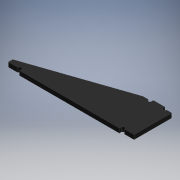
# Autodesk Inventor part: 前腕_サブフレーム_1_1
Saved by Autodesk Inventor 2018 (Build 220112000, 112)
## iProperties
Created: 2016-05-04
Part Number: 前腕_サブフレーム_1_1
Material: アセタール樹脂、黒
Document SubType Name: Modeling
Designer: hiroaki
Density: 1.425 g/cm^3
Appearance: 滑らか - 黒
Mass: 16.6655 g
Surface Area: 81.5563 cm^2
Volume: 11.6951 cm^3
Author: hiroaki
Autodesk Inventor part; units mm, degrees
ref_plane "YZ Plane" through (0, 0, 0) normal (1, 0, 0) x (0, 1, 0)
ref_plane "XZ Plane" through (0, 0, 0) normal (0, 1, 0) x (-1, 0, 0)
ref_plane "XY Plane" through (0, 0, 0) normal (0, 0, 1) x (1, 0, 0)
sketch "スケッチ1" plane through (0, 0, 0) normal (0, 0, 1) x (1, 0, 0)
  line L0 (-72.5, -21.65) -> (72.5, -21.65) construction
  line L1 (72.5, -21.65) -> (72.5, 21.65) construction
  line L2 (72.5, 21.65) -> (-72.5, 21.65) construction
  line L3 (-72.5, 21.65) -> (-72.5, -21.65) construction
  line L4 (-72.5, -21.65) -> (72.5, 21.65) construction
  line L5 (72.5, -21.65) -> (-72.5, 21.65) construction
  line L6 (-67.5, 21.65) -> (-67.5, -21.65) construction
  line L7 (0, 0) -> (0, 21.65) construction
  line L8 (0, 0) -> (-72.5, 0) construction
  line L9 (67.5, 21.65) -> (67.5, -21.65) construction
  line L10 (-72.5, -21.65) -> (-61.6, -21.65)
  line L11 (49.5, 21.65) -> (49.5, 23.65)
  line L12 (49.5, 23.65) -> (62.5, 23.65)
  line L13 (62.5, 23.65) -> (62.5, 21.65)
  line L14 (66.6, 21.65) -> (72.5, 21.65)
  line L15 (72.5, 21.65) -> (72.5, -21.65)
  line L16 (72.5, -21.65) -> (61.6, -21.65)
  line L17 (-57.5, -21.65) -> (-57.5, -23.65)
  line L18 (-57.5, -23.65) -> (57.5, -23.65)
  line L19 (57.5, -23.65) -> (57.5, -21.65)
  arc A0 (45.4, 21.65) -> (49.5, 21.65) centre (47.45, 21.65) ccw
  arc A1 (62.5, 21.65) -> (66.6, 21.65) centre (64.55, 21.65) ccw
  arc A2 (-57.5, -21.65) -> (-61.6, -21.65) centre (-59.55, -21.65) ccw
  arc A3 (61.6, -21.65) -> (57.5, -21.65) centre (59.55, -21.65) ccw
  line L20 (-72.5, -21.65) -> (-72.5, -16.65)
  line L21 (-72.5, -16.65) -> (39.5, 21.65)
  line L22 (45.4, 21.65) -> (39.5, 21.65)
  line L23 (66.95, 24.476) -> (70.05, 24.476) construction
  line L24 (70.05, 24.476) -> (70.05, 13.3235) construction
  line L25 (70.05, 13.3235) -> (66.95, 13.3235) construction
  line L26 (66.95, 13.3235) -> (66.95, 24.476) construction
  line L27 (68.5, 24.476) -> (68.5, 13.3235) construction
  line L28 (41.95, 24.476) -> (45.05, 24.476) construction
  line L29 (45.05, 24.476) -> (45.05, 13.9945) construction
  line L30 (45.05, 13.9945) -> (41.95, 13.9945) construction
  line L31 (41.95, 13.9945) -> (41.95, 24.476) construction
  line L32 (43.5, 24.476) -> (43.5, 13.9945) construction
  dimension "d16" = 5
  dimension "d20" = 43.3
  dimension "d40" = 135
  dimension "d41" = 10
  dimension "d42" = 2.05
  dimension "d43" = 2
  dimension "d44" = 5
  dimension "d45" = 10
  dimension "d46" = 10
  dimension "d48" = 3.1
  dimension "d50" = 4
  dimension "d51" = 25
  dimension "d52" = 3.1
  dimension "d62" = 6
  dimension "d63" = 6
  constraints: 66 end point, 11 perpendicular, 8 midpoint, 8 point on circle, 6 parallel, 6 point on line, 5 collinear, 4 centre point, 4 horizontal, 4 horizontal alignment, 3 equal radius, 3 tangent, 2 symmetric about line, 2 vertical, 3 other
  measures "d16" distance between parallel lines of L3 L6
  measures "d20" distance of L2.end L0.start
  measures "d40" distance between parallel lines of L9 L6
  measures "d41" distance between parallel lines of L6 L17
  measures "d42" radius of A2
  measures "d43" distance between parallel lines of L0 L18
  measures "d44" distance from line of L10 L20.end
  measures "d45" distance between parallel lines of L1 L13
  measures "d46" distance from line of L21.end L11
  measures "d48" distance of L23.start L23.end
  measures "d50" distance between parallel lines of L1 L27
  measures "d51" distance between parallel lines of L27 L32
  measures "d52" distance of L28.start L28.end
  measures "d62" distance between parallel lines of L13 L27
  measures "d63" distance between parallel lines of L32 L11
extrude "押し出し1" add sketch "スケッチ1" along normal blind 2.5
mirror "ミラー1" about plane through (8.3734, -6.8299, 0) normal (0, 0, -1) of "押し出し1"
equation "\"d16\" = d4"
equation "\"d40\" = d6"
equation "\"d41\" = d3"
equation "\"d46\" = d45"
equation "\"d63\" = d62"
equation "\"d4\" = 5"
equation "\"d6\" = 135"
equation "\"d3\" = 10"
